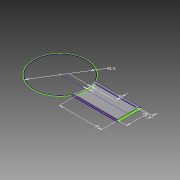
# Autodesk Inventor part: Pump lid MM0312
Saved by Autodesk Inventor 2013 SP2 (Build 170200200, 200)
## iProperties
Created: 2015-07-01
Part Number: Pump lid MM0312
Material: Generic
Document SubType Name: Modeling
Designer: kthorn
Density: 1 g/cm^3
Author: kthorn
Autodesk Inventor part; units mm, degrees
ref_plane "YZ Plane" through (0, 0, 0) normal (1, 0, 0) x (0, 1, 0)
ref_plane "XZ Plane" through (0, 0, 0) normal (0, 1, 0) x (-1, 0, 0)
ref_plane "XY Plane" through (0, 0, 0) normal (0, 0, 1) x (1, 0, 0)
sketch "Sketch1" plane through (0, 0, 0) normal (0, 0, 1) x (1, 0, 0)
  circle A0 centre (0, 0) radius 45.75
  circle A1 centre (0, 0) radius 46.75
  line L0 (45.75, -0.0157) -> (46.75, -0.0157) construction
  line L1 (42.7149, 19) -> (121.75, 19)
  line L2 (121.75, 19) -> (121.75, -19)
  line L3 (121.75, -19) -> (42.7149, -19)
  line L4 (41.768, 21) -> (123.75, 21)
  line L5 (123.75, 21) -> (123.75, -21)
  line L6 (123.75, -21) -> (41.768, -21)
  line L7 (82.759, 21) -> (82.759, 19) construction
  line L8 (121.75, 0) -> (123.75, 0) construction
  line L9 (98.0367, -19) -> (98.0367, -21) construction
  line L10 (0, 0) -> (121.75, 0) construction
  line L11 (41.768, 21) -> (40.6456, 21)
  line L12 (41.768, -21) -> (40.6456, -21)
  line L13 (45.6899, 17) -> (119.75, 17)
  line L14 (119.75, 17) -> (119.75, -17)
  arc A2 (44.895, -19) -> (44.895, 19) centre (0, 0) ccw
  line L15 (119.75, -17) -> (45.6899, -17)
  dimension "d0" = 91.5
  dimension "d2" = 1
  dimension "d3" = 75
  dimension "d4" = 38
  dimension "d5" = 2
  dimension "d62" = 2
  dimension "d63" = 2
  constraints: 32 end point, 12 point on circle, 6 perpendicular, 5 parallel, 5 point on line, 3 centre point, 3 horizontal, 3 midpoint, 2 equal length, 1 coincident
  measures "d0" diameter of A0
  measures "d2" distance of L0.end L0.start
  measures "d3" distance from line of L2 L0.end
  measures "d4" distance of L1.end L2.end
  measures "d5" distance of L7.start L7.end
  measures "d62" distance between parallel lines of L1 L13
  measures "d63" radial gap between concentric circles of A1 A2
extrude "Extrusion13" add sketch "Sketch1" against normal blind 2 contours A0 L11 A1 L12 | L4 L5 L6 A1 L3 L2 L1 | L1 A2 L3 A1 | L1 L2 L3 A2 L15 L14 L13 | L13 L14 L15 A2 picked at (42.2726, -18.1004)
extrude "Extrusion14" add sketch "Sketch1" along normal blind 2 contours L1 A2 L3 A1 | L1 L2 L3 A2 L15 L14 L13
body "Solid2"
